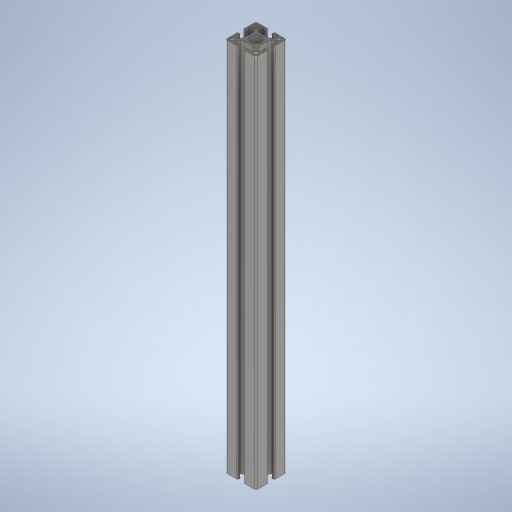
# Autodesk Inventor part: Perfil aluminio
Saved by Autodesk Inventor 2023 (Build 270158000, 158)
## iProperties
Created: 2023-04-11
Part Number: Perfil aluminio
Material: Alumínio 6061
Document SubType Name: Sheet Metal
Designer: Mateus PC
Density: 2.7 g/cm^3
Sheet Metal Rule: Default_mm
Appearance: Semipolido
Author: Mateus PC
Autodesk Inventor part; units mm, degrees
ref_plane "YZ Plane" through (0, 0, 0) normal (1, 0, 0) x (0, 1, 0)
ref_plane "XZ Plane" through (0, 0, 0) normal (0, 1, 0) x (-1, 0, 0)
ref_plane "XY Plane" through (0, 0, 0) normal (0, 0, 1) x (1, 0, 0)
sketch "Esboço1" plane through (0, 0, 0) normal (0, 1, 0) x (-1, 0, 0)
  line L0 (0, 0) -> (15.905, 0)
  line L1 (15.905, 0) -> (15.905, -3.81)
  line L2 (15.905, -3.81) -> (12.81, -3.81)
  line L3 (12.81, -3.81) -> (12.81, -2)
  line L4 (12.81, -2) -> (9, -2)
  line L5 (31, -2) -> (27.19, -2)
  line L6 (27.19, -2) -> (27.19, -3.81)
  line L7 (27.19, -3.81) -> (24.095, -3.81)
  line L8 (24.095, -3.81) -> (24.095, 0)
  line L9 (24.095, 0) -> (40, 0)
  line L10 (40, 0) -> (40, -15.905)
  line L11 (40, -15.905) -> (36.19, -15.905)
  line L12 (36.19, -15.905) -> (36.19, -12.81)
  line L13 (36.19, -12.81) -> (38, -12.81)
  line L14 (38, -12.81) -> (38, -9)
  line L15 (38, -31) -> (38, -27.19)
  line L16 (38, -27.19) -> (36.19, -27.19)
  line L17 (36.19, -27.19) -> (36.19, -24.095)
  line L18 (36.19, -24.095) -> (40, -24.095)
  line L19 (40, -24.095) -> (40, -40)
  line L20 (40, -40) -> (24.095, -40)
  line L21 (24.095, -40) -> (24.095, -36.19)
  line L22 (24.095, -36.19) -> (27.19, -36.19)
  line L23 (27.19, -36.19) -> (27.19, -38)
  line L24 (27.19, -38) -> (31, -38)
  line L25 (9, -38) -> (12.81, -38)
  line L26 (12.81, -38) -> (12.81, -36.19)
  line L27 (12.81, -36.19) -> (15.905, -36.19)
  line L28 (15.905, -36.19) -> (15.905, -40)
  line L29 (15.905, -40) -> (0, -40)
  line L30 (0, -40) -> (0, -24.095)
  line L31 (0, -24.095) -> (3.81, -24.095)
  line L32 (3.81, -24.095) -> (3.81, -27.19)
  line L33 (3.81, -27.19) -> (2, -27.19)
  line L34 (2, -27.19) -> (2, -31)
  line L35 (2, -9) -> (2, -12.81)
  line L36 (2, -12.81) -> (3.81, -12.81)
  line L37 (3.81, -12.81) -> (3.81, -15.905)
  line L38 (3.81, -15.905) -> (0, -15.905)
  line L39 (0, -15.905) -> (0, 0)
  line L40 (38, -9) -> (33.5, -9)
  line L41 (33.5, -9) -> (30, -12.5)
  line L42 (30, -12.5) -> (30, -27.5)
  line L43 (30, -27.5) -> (33.5, -31)
  line L44 (33.5, -31) -> (38, -31)
  line L45 (31, -2) -> (31, -6.5)
  line L46 (31, -6.5) -> (27.5, -10)
  line L47 (27.5, -10) -> (12.5, -10)
  line L48 (12.5, -10) -> (9, -6.5)
  line L49 (9, -6.5) -> (9, -2)
  line L50 (2, -9) -> (6.5, -9)
  line L51 (6.5, -9) -> (10, -12.5)
  line L52 (10, -12.5) -> (10, -27.5)
  line L53 (10, -27.5) -> (6.5, -31)
  line L54 (6.5, -31) -> (2, -31)
  line L55 (9, -38) -> (9, -33.5)
  line L56 (9, -33.5) -> (12.5, -30)
  line L57 (12.5, -30) -> (27.5, -30)
  line L58 (27.5, -30) -> (31, -33.5)
  line L59 (31, -33.5) -> (31, -38)
  dimension "d11" = 15.905
  dimension "d12" = 40
  dimension "d13" = 3.81
  dimension "d14" = 22
  dimension "d15" = 20
  dimension "d17" = 3.81
  dimension "d18" = 2
  dimension "d19" = 15
  constraints: 120 end point, 48 equal length, 37 perpendicular, 9 point on line, 8 parallel, 4 horizontal, 4 vertical
  measures "d11" distance of L19.end L20.end
  measures "d12" distance of L29.end L19.end
  measures "d13" distance of L20.end L21.end
  measures "d14" distance of L25.start L24.end
  measures "d15" distance of L52.end L42.end
  measures "d17" distance of L23.end L24.end
  measures "d18" distance from line of L20 L23.end
  measures "d19" distance of L52.end L51.end
extrude "Extrusão1" add sketch "Esboço1" along normal blind 494
sketch "Esboço3" plane through (0, 494, 0) normal (0, 1, 0) x (1, 0, 0)
  point P0 (0, 0)
fillet "Arredondamento1" radius 2 4 edges at (-40, 247, -40) (-40, 247, 0) (0, 247, -40) (0, 247, 0)
fillet "Arredondamento2" radius 1 38 edges at (-38, 247, -31) (-36.19, 247, -27.19) (-36.19, 247, -24.095) (-38, 247, -27.19) (-31, 247, -38) (-24.095, 247, -36.19) (-24.095, 247, -40) (-15.905, 247, -36.19) (-12.81, 247, -36.19) (-12.81, 247, -38) (-27.19, 247, -36.19) (-27.19, 247, -38) (-40, 247, -15.905) (-36.19, 247, -15.905) (-36.19, 247, -12.81) (-38, 247, -9) (-38, 247, -12.81) (-24.095, 247, 0) (-24.095, 247, -3.81) (-27.19, 247, -3.81) (-27.19, 247, -2) (-9, 247, -2) (-15.905, 247, -3.81) (-12.81, 247, -3.81) (-3.81, 247, -12.81) (-3.81, 247, -15.905) (0, 247, -15.905) (-2, 247, -27.19) (-3.81, 247, -27.19) (-3.81, 247, -24.095) (-15.905, 247, -40) (0, 247, -24.095) (-12.81, 247, -2) (-15.905, 247, 0) (-2, 247, -9) (-2, 247, -31) (-9, 247, -38) (-31, 247, -2)
fillet "Arredondamento3" radius 3 8 edges at (-9, 247, -33.5) (-33.5, 247, -9) (-31, 247, -33.5) (-31, 247, -6.5) (-9, 247, -6.5) (-6.5, 247, -9) (-6.5, 247, -31) (-33.5, 247, -31)
fillet "Arredondamento4" radius 6 8 edges at (-30, 247, -27.5) (-30, 247, -12.5) (-27.5, 247, -30) (-12.5, 247, -30) (-10, 247, -12.5) (-10, 247, -27.5) (-27.5, 247, -10) (-12.5, 247, -10)
sketch "Esboço4" plane through (0, 0, 0) normal (0, -1, 0) x (1, 0, 0)
  circle A0 centre (-20, -20) radius 7
  line L0 (-10, -14.9853) -> (-10, -25.0147) projected
  line L1 (-25.0147, -10) -> (-14.9853, -10) projected
  arc A1 (-40, -38) -> (-38, -40) centre (-38, -38) ccw projected
  line L2 (-40, -38) -> (-40, -24.095) projected
  line L3 (-40, -24.095) -> (-37.19, -24.095) projected
  arc A2 (-36.19, -25.095) -> (-37.19, -24.095) centre (-37.19, -25.095) ccw projected
  line L4 (-36.19, -25.095) -> (-36.19, -26.19) projected
  arc A3 (-37.095, -27.1855) -> (-36.19, -26.19) centre (-37.19, -26.19) ccw projected
  line L5 (-38, -28.181) -> (-38, -30) projected
  arc A4 (-38, -30) -> (-37, -31) centre (-37, -30) ccw projected
  line L6 (-37, -31) -> (-34.7426, -31) projected
  arc A5 (-34.7426, -31) -> (-32.6213, -30.1213) centre (-34.7426, -28) ccw projected
  line L7 (-32.6213, -30.1213) -> (-31.7574, -29.2574) projected
  arc A6 (-31.7574, -29.2574) -> (-30, -25.0147) centre (-36, -25.0147) ccw projected
  line L8 (-30, -25.0147) -> (-30, -14.9853) projected
  arc A7 (-30, -14.9853) -> (-31.7574, -10.7426) centre (-36, -14.9853) ccw projected
  line L9 (-31.7574, -10.7426) -> (-32.6213, -9.8787) projected
  arc A8 (-32.6213, -9.8787) -> (-34.7426, -9) centre (-34.7426, -12) ccw projected
  line L10 (-34.7426, -9) -> (-37, -9) projected
  arc A9 (-37, -9) -> (-38, -10) centre (-37, -10) ccw projected
  line L11 (-38, -10) -> (-38, -11.819) projected
  arc A10 (-36.19, -13.81) -> (-37.095, -12.8145) centre (-37.19, -13.81) ccw projected
  line L12 (-36.19, -13.81) -> (-36.19, -14.905) projected
  arc A11 (-37.19, -15.905) -> (-36.19, -14.905) centre (-37.19, -14.905) ccw projected
  line L13 (-37.19, -15.905) -> (-39, -15.905) projected
  arc A12 (-40, -14.905) -> (-39, -15.905) centre (-39, -14.905) ccw projected
  line L14 (-40, -14.905) -> (-40, -2) projected
  arc A13 (-38, 0) -> (-40, -2) centre (-38, -2) ccw projected
  line L15 (-38, 0) -> (-25.095, 0) projected
  arc A14 (-24.095, -1) -> (-25.095, 0) centre (-25.095, -1) ccw projected
  line L16 (-24.095, -1) -> (-24.095, -2.81) projected
  arc A15 (-25.095, -3.81) -> (-24.095, -2.81) centre (-25.095, -2.81) ccw projected
  line L17 (-25.095, -3.81) -> (-26.19, -3.81) projected
  arc A16 (-27.1855, -2.905) -> (-26.19, -3.81) centre (-26.19, -2.81) ccw projected
  line L18 (-28.181, -2) -> (-30, -2) projected
  arc A17 (-30, -2) -> (-31, -3) centre (-30, -3) ccw projected
  line L19 (-31, -3) -> (-31, -5.2574) projected
  arc A18 (-31, -5.2574) -> (-30.1213, -7.3787) centre (-28, -5.2574) ccw projected
  line L20 (-30.1213, -7.3787) -> (-29.2574, -8.2426) projected
  arc A19 (-29.2574, -8.2426) -> (-25.0147, -10) centre (-25.0147, -4) ccw projected
  line L21 (-25.0147, -10) -> (-14.9853, -10) projected
  arc A20 (-14.9853, -10) -> (-10.7426, -8.2426) centre (-14.9853, -4) ccw projected
  line L22 (-10.7426, -8.2426) -> (-9.8787, -7.3787) projected
  arc A21 (-9.8787, -7.3787) -> (-9, -5.2574) centre (-12, -5.2574) ccw projected
  line L23 (-9, -5.2574) -> (-9, -3) projected
  arc A22 (-9, -3) -> (-10, -2) centre (-10, -3) ccw projected
  line L24 (-10, -2) -> (-11.819, -2) projected
  arc A23 (-13.81, -3.81) -> (-12.8145, -2.905) centre (-13.81, -2.81) ccw projected
  line L25 (-13.81, -3.81) -> (-14.905, -3.81) projected
  arc A24 (-15.905, -2.81) -> (-14.905, -3.81) centre (-14.905, -2.81) ccw projected
  line L26 (-15.905, -2.81) -> (-15.905, -1) projected
  arc A25 (-14.905, 0) -> (-15.905, -1) centre (-14.905, -1) ccw projected
  line L27 (-14.905, 0) -> (-2, 0) projected
  arc A26 (0, -2) -> (-2, 0) centre (-2, -2) ccw projected
  line L28 (0, -2) -> (0, -14.905) projected
  arc A27 (-1, -15.905) -> (0, -14.905) centre (-1, -14.905) ccw projected
  line L29 (-1, -15.905) -> (-2.81, -15.905) projected
  arc A28 (-3.81, -14.905) -> (-2.81, -15.905) centre (-2.81, -14.905) ccw projected
  line L30 (-3.81, -14.905) -> (-3.81, -13.81) projected
  arc A29 (-2.81, -12.81) -> (-3.81, -13.81) centre (-2.81, -13.81) ccw projected
  line L31 (-2.81, -12.81) -> (-2, -12.81) projected
  line L32 (-2, -12.81) -> (-2, -10) projected
  arc A30 (-2, -10) -> (-3, -9) centre (-3, -10) ccw projected
  line L33 (-3, -9) -> (-5.2574, -9) projected
  arc A31 (-5.2574, -9) -> (-7.3787, -9.8787) centre (-5.2574, -12) ccw projected
  line L34 (-7.3787, -9.8787) -> (-8.2426, -10.7426) projected
  arc A32 (-8.2426, -10.7426) -> (-10, -14.9853) centre (-4, -14.9853) ccw projected
  line L35 (-10, -14.9853) -> (-10, -25.0147) projected
  arc A33 (-10, -25.0147) -> (-8.2426, -29.2574) centre (-4, -25.0147) ccw projected
  line L36 (-8.2426, -29.2574) -> (-7.3787, -30.1213) projected
  arc A34 (-7.3787, -30.1213) -> (-5.2574, -31) centre (-5.2574, -28) ccw projected
  line L37 (-5.2574, -31) -> (-3, -31) projected
  arc A35 (-3, -31) -> (-2, -30) centre (-3, -30) ccw projected
  line L38 (-2, -30) -> (-2, -28.19) projected
  arc A36 (-2, -28.19) -> (-2.905, -27.1945) centre (-3, -28.19) ccw projected
  line L39 (-3.81, -26.199) -> (-3.81, -25.095) projected
  arc A37 (-2.81, -24.095) -> (-3.81, -25.095) centre (-2.81, -25.095) ccw projected
  line L40 (-2.81, -24.095) -> (-1, -24.095) projected
  arc A38 (0, -25.095) -> (-1, -24.095) centre (-1, -25.095) ccw projected
  line L41 (0, -25.095) -> (0, -38) projected
  arc A39 (-2, -40) -> (0, -38) centre (-2, -38) ccw projected
  line L42 (-2, -40) -> (-14.905, -40) projected
  arc A40 (-15.905, -39) -> (-14.905, -40) centre (-14.905, -39) ccw projected
  line L43 (-15.905, -39) -> (-15.905, -37.19) projected
  arc A41 (-14.905, -36.19) -> (-15.905, -37.19) centre (-14.905, -37.19) ccw projected
  line L44 (-14.905, -36.19) -> (-13.81, -36.19) projected
  arc A42 (-12.8145, -37.095) -> (-13.81, -36.19) centre (-13.81, -37.19) ccw projected
  line L45 (-11.819, -38) -> (-10, -38) projected
  arc A43 (-10, -38) -> (-9, -37) centre (-10, -37) ccw projected
  line L46 (-9, -37) -> (-9, -34.7426) projected
  arc A44 (-9, -34.7426) -> (-9.8787, -32.6213) centre (-12, -34.7426) ccw projected
  line L47 (-9.8787, -32.6213) -> (-10.7426, -31.7574) projected
  arc A45 (-10.7426, -31.7574) -> (-14.9853, -30) centre (-14.9853, -36) ccw projected
  line L48 (-14.9853, -30) -> (-25.0147, -30) projected
  arc A46 (-25.0147, -30) -> (-29.2574, -31.7574) centre (-25.0147, -36) ccw projected
  line L49 (-29.2574, -31.7574) -> (-30.1213, -32.6213) projected
  arc A47 (-30.1213, -32.6213) -> (-31, -34.7426) centre (-28, -34.7426) ccw projected
  line L50 (-31, -34.7426) -> (-31, -37) projected
  arc A48 (-31, -37) -> (-30, -38) centre (-30, -37) ccw projected
  line L51 (-30, -38) -> (-28.181, -38) projected
  arc A49 (-26.19, -36.19) -> (-27.1855, -37.095) centre (-26.19, -37.19) ccw projected
  line L52 (-26.19, -36.19) -> (-25.095, -36.19) projected
  arc A50 (-24.095, -37.19) -> (-25.095, -36.19) centre (-25.095, -37.19) ccw projected
  line L53 (-24.095, -37.19) -> (-24.095, -39) projected
  arc A51 (-25.095, -40) -> (-24.095, -39) centre (-25.095, -39) ccw projected
  line L54 (-25.095, -40) -> (-38, -40) projected
  circle A52 centre (-4.5, -4.5) radius 2.5
  circle A53 centre (-4.5, -35.5) radius 2.5
  circle A54 centre (-35.5, -35.5) radius 2.5
  circle A55 centre (-35.5, -4.5) radius 2.5
  arc A56 (-37.095, -27.1855) -> (-38, -28.181) centre (-37, -28.181) ccw projected
  arc A57 (-38, -11.819) -> (-37.095, -12.8145) centre (-37, -11.819) ccw projected
  arc A58 (-27.1855, -2.905) -> (-28.181, -2) centre (-28.181, -3) ccw projected
  arc A59 (-11.819, -2) -> (-12.8145, -2.905) centre (-11.819, -3) ccw projected
  arc A60 (-3.81, -26.199) -> (-2.905, -27.1945) centre (-2.81, -26.199) ccw projected
  arc A61 (-12.8145, -37.095) -> (-11.819, -38) centre (-11.819, -37) ccw projected
  arc A62 (-28.181, -38) -> (-27.1855, -37.095) centre (-28.181, -37) ccw projected
  point P0 (0, 0)
  point P1 (-10, -20)
  point P2 (-20, -10)
  dimension "d26" = 14
  dimension "d27" = 0
  dimension "d28" = 0
  dimension "d29" = 40
  dimension "d30" = 5
  dimension "d31" = 5
  dimension "d32" = 5
  dimension "d33" = 5
  dimension "d34" = 31
  dimension "d35" = 4.5
  dimension "d36" = 31
  dimension "d37" = 4.5
  dimension "d38" = 31
  dimension "d39" = 31
  dimension "d40" = 4.5
  dimension "d41" = 4.5
  constraints: 5 centre point, 2 midpoint
  measures "d26" diameter of A0
  measures "d27" vertical distance of A0.centre point (-10, -20)
  measures "d28" horizontal distance of point (-20, -10) A0.centre
  measures "d29" distance between parallel lines of L42 L27
  measures "d30" diameter of A52
  measures "d31" diameter of A53
  measures "d32" diameter of A54
  measures "d33" diameter of A55
  measures "d34" distance of A53.centre A52.centre
  measures "d35" distance from line of L42 A53.centre
  measures "d36" distance of A54.centre A53.centre
  measures "d37" distance from line of L41 A53.centre
  measures "d38" distance of A55.centre A54.centre
  measures "d39" distance of A52.centre A55.centre
  measures "d40" distance from line of L28 A52.centre
  measures "d41" distance from line of L15 A55.centre
extrude "Extrusão2" cut sketch "Esboço4" against normal through all contours A0 | A52 | A53 | A54 | A55
equation "\"d17\" = d13"
equation "\"d35\" = -0.5 * d34 + 0.5 * d29"
equation "\"d36\" = d34"
equation "\"d37\" = d35"
equation "\"d38\" = d36"
equation "\"d39\" = d36"
equation "\"d40\" = d37"
equation "\"d41\" = d35"
equation "\"Raio_vergadura\" = Espessura"
equation "\"Largura_alívio_de_vergadura\" = Espessura"
equation "\"Profundidade_alívio_de_vergadura\" = 0.5 * Espessura"
equation "\"Tamanho_alívio_de_dobra\" = 4 * Espessura"
equation "\"Remanescente_mínimo\" = 2 * Espessura"
equation "\"Raiodetransição\" = Raio_vergadura"
equation "\"Tamanho_de_raio_de_Jacobi\" = Raio_vergadura"
equation "\"TamanhoFolga\" = Espessura"
equation "\"Espessura\" = 0.5"
